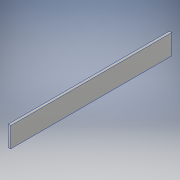
# Autodesk Inventor part: CLB_091_ClimberSupportBar
Saved by Autodesk Inventor 2018 (Build 220112000, 112)
## iProperties
Created: 2020-03-03
Part Number: CLB_091_ClimberSupportBar
Material: Aluminum 6061
Document SubType Name: Modeling
Designer: Cooper
Density: 2.7 g/cm^3
Appearance: Aluminum - Flat
Author: Cooper
Autodesk Inventor part; units mm, degrees
ref_plane "YZ Plane" through (0, 0, 0) normal (1, 0, 0) x (0, 1, 0)
ref_plane "XZ Plane" through (0, 0, 0) normal (0, 1, 0) x (-1, 0, 0)
ref_plane "XY Plane" through (0, 0, 0) normal (0, 0, 1) x (1, 0, 0)
sketch "Sketch1" plane through (0, 0, 0) normal (0, 0, 1) x (1, 0, 0)
  line L0 (0, 0) -> (3.175, 0)
  line L1 (3.175, 0) -> (3.175, 25.4)
  line L2 (3.175, 25.4) -> (0, 25.4)
  line L3 (0, 25.4) -> (0, 0)
  dimension "d0" = 3.175
  dimension "d1" = 25.4
  constraints: 8 end point, 2 parallel, 1 horizontal, 1 perpendicular
  measures "d0" distance of L0.start L0.end
  measures "d1" distance of L2.end L0.start
extrude "Extrusion1" add sketch "Sketch1" along normal blind 203.2
body "Solid1"
